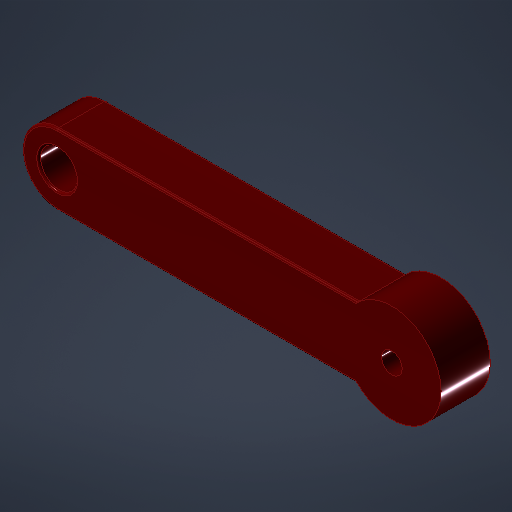
# Autodesk Inventor part: Arm Link Lower
Saved by Autodesk Inventor 2026.2 (Build 302298010, 298A)
## iProperties
Created: 2026-05-30
Part Number: Arm Link Lower
Material: Generic
Document SubType Name: Modeling
Designer: yassi
Density: 1 g/cm^3
Appearance: Light Red
Author: yassi
## iProperties of the stored document Arm Link Lower_3DPrint.ipt
Created: 2026-06-01
Part Number: Arm Link Lower_3DPrint
Material: Generic
Document SubType Name: Modeling
Designer: yassi
Density: 1 g/cm^3
Appearance: Default
Author: yassi
Autodesk Inventor part; units mm, degrees
ref_plane "YZ Plane" through (0, 0, 0) normal (1, 0, 0) x (0, 1, 0)
ref_plane "XZ Plane" through (0, 0, 0) normal (0, 1, 0) x (-1, 0, 0)
ref_plane "XY Plane" through (0, 0, 0) normal (0, 0, 1) x (1, 0, 0)
sketch "Sketch1" plane through (0, 0, 0) normal (0, 0, 1) x (1, 0, 0)
  circle A0 centre (0, 0) radius 4.7
  arc A1 (0, 9) -> (0, -9) centre (0, 0) ccw
  circle A2 centre (85, 0) radius 2.65
  arc A3 (76.3253, -9) -> (76.3253, 9) centre (85, 0) ccw
  line L0 (0, 9) -> (76.3253, 9)
  line L1 (0, -9) -> (76.3253, -9)
  dimension "d0" = 9.4
  dimension "d1" = 18
  dimension "d3" = 5.3
  dimension "d4" = 25
  constraints: 4 centre point, 4 end point, 4 point on circle, 3 coincident, 1 horizontal, 1 parallel, 1 tangent
  measures "d0" diameter of A0
  measures "d1" diameter of A1
  measures "d3" diameter of A2
  measures "d4" diameter of A3
extrude "Extrusion1" add sketch "Sketch1" along normal blind 12.5
fillet "Fillet1" radius 0.5 8 edges at (-4.7, 0, 0) (-9, 0, 0) (38.1627, 9, 0) (38.1627, -9, 0) (-9, 0, 12.5) (38.1627, 9, 12.5) (38.1627, -9, 12.5) (-4.7, 0, 12.5)
body "Solid1"
